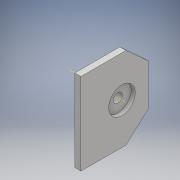
# Autodesk Inventor part: percuteur
Saved by Autodesk Inventor 2017 (Build 210142000, 142)
## iProperties
Part Number: percuteur
Material: Générique
Document SubType Name: Modeling
Designer: Thomas
Density: 1 g/cm^3
Appearance: Par défaut
Author: Thomas
Autodesk Inventor part; units mm, degrees
ref_plane "YZ Plane" through (0, 0, 0) normal (1, 0, 0) x (0, 1, 0)
ref_plane "XZ Plane" through (0, 0, 0) normal (0, 1, 0) x (-1, 0, 0)
ref_plane "XY Plane" through (0, 0, 0) normal (0, 0, 1) x (1, 0, 0)
sketch "Esquisse1" plane through (0, 0, 0) normal (1, 0, 0) x (0, 1, 0)
  circle A0 centre (0, 0) radius 5.25
  circle A1 centre (0, 0) radius 7
  dimension "d0" = 10.5
  dimension "d1" = 14
  constraints: 2 centre point, 2 coincident
  measures "d0" diameter of A0
  measures "d1" diameter of A1
extrude "Extrusion1" add sketch "Esquisse1" along normal blind 10
sketch "Esquisse2" plane through (10, 0, 0) normal (1, 0, 0) x (0, 0, -1)
  line L0 (20, -20) -> (-20, 20) construction
  line L1 (-20, -20) -> (20, 20) construction
  circle A0 centre (0, 0) radius 17.5 construction
  line L2 (0, 0) -> (0, 13) construction
  line L3 (0, 13) -> (10, 13)
  line L4 (10, 13) -> (-10, 13)
  line L5 (0, 0) -> (0, -20) construction
  line L6 (0, -20) -> (20, -20)
  line L7 (20, -20) -> (-20, -20)
  line L8 (-20, -20) -> (-20, 2)
  line L9 (20, -20) -> (20, 2)
  line L10 (20, 2) -> (10, 13)
  line L11 (-10, 13) -> (-20, 2)
  dimension "d41" = 35
  dimension "d44" = 13
  dimension "d45" = 10
  dimension "d46" = 20
  dimension "d47" = 20
  dimension "d48" = 20
  dimension "d49" = 22
  dimension "d50" = 14.8661
  dimension "d51" = 14.8661
  constraints: 24 end point, 3 point on line, 3 vertical, 2 horizontal, 2 midpoint, 1 centre point, 1 coincident, 1 perpendicular
  measures "d41" diameter of A0
  measures "d44" distance of L2.start L2.end
  measures "d45" distance of L2.end L3.end
  measures "d46" distance of L3.end L4.end
  measures "d47" distance of L2.start L5.end
  measures "d48" distance of L5.end L0.start
  measures "d49" distance of L7.end L8.end
  measures "d50" distance of L9.end L3.end
  measures "d51" distance of L4.end L8.end
extrude "Extrusion2" add sketch "Esquisse2" along normal blind 3
sketch "Esquisse7" plane through (13, 0, 0) normal (1, 0, 0) x (0, 0, -1)
  circle A0 centre (0, 0) radius 2.25
  dimension "d25" = 4.5
  constraints: 1 centre point, 1 coincident
  measures "d25" diameter of A0
extrude "Extrusion7" cut sketch "Esquisse7" against normal blind 59.75
sketch "Esquisse12" plane through (0, 0, 0) normal (-1, 0, 0) x (0, 0, 1)
  circle A0 centre (0, 0) radius 5.25 projected
  circle A1 centre (0, 0) radius 7 projected
extrude "Extrusion10" cut sketch "Esquisse12" against normal blind 5
sketch "Esquisse13" plane through (13, 0, 0) normal (1, 0, 0) x (0, 0, -1)
  circle A0 centre (0, 0) radius 6.5
  dimension "d52" = 13
  constraints: 1 centre point, 1 coincident
  measures "d52" diameter of A0
extrude "Extrusion11" cut sketch "Esquisse13" against normal blind 2
sketch "Esquisse14" plane through (10, 0, 0) normal (-1, 0, 0) x (0, 0, 1)
  circle A0 centre (0, 0) radius 2.25 projected
  circle A1 centre (0, 0) radius 5.25 projected
extrude "Extrusion12" add sketch "Esquisse14" along normal blind 3
